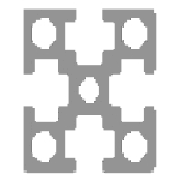
# Autodesk Inventor part: r150
Saved by Autodesk Inventor 2018 (Build 220112000, 112)
## iProperties
_CCFamilyMember: 1
_CCFamilyDisplayName: MISUMI_AFS - MISUMI Frame Family
_FrameMemberDoc: Frame Member File
_Version: 15.0.0
_GetPNFromCC: 1
Created: 2016-02-19
Part Number: r150
Material: アルミニウム 6061
Description: MISUMI Frame Family
Document SubType Name: Modeling
Standard: 名称未設定
Designer: gisen
Language: ja-JP
Size Designation: (名称未設定 1)
Categories: <MemberInstance><Categories><Category DisplayName="形鋼" InternalName="089c4875-fa83-4c05-b084-43b9cc11f5ed" Mnemonic="GRDR"><CategoryParameter DisplayName="長さ単位ごとの質量" InternalName="0bb95a10-148f-4027-a459-38d7b056702a" Mnemonic="shpmass"/><CategoryParameter DisplayName="断面積" InternalName="1ff91680-64b0-4202-b9a3-7fd3f94bba3b" Mnemonic="secarea"/><CategoryParameter DisplayName="回転半径(x)" InternalName="25778675-03e9-40c1-b6a8-4a9ed693320d" Mnemonic="gyrradx"/><CategoryParameter DisplayName="横弾性係数" InternalName="26c1ec35-5026-4c63-ad0a-751cf684a536" Mnemonic="torrigmod"/><CategoryParameter DisplayName="重心 X-X 間の距離" InternalName="26c9bdb8-9c79-4b4f-a92e-8e197583c9c4" Mnemonic="grcendistX"/><CategoryParameter DisplayName="レガシー メンバ ID" InternalName="340afe4f-75d7-48d3-ab7d-943f3c3da468" Mnemonic="LegacyMemberID"/><CategoryParameter DisplayName="基準長さ" InternalName="42e34263-8f20-4d0e-ad48-bf1385b87c24" Mnemonic="shplen"/><CategoryParameter DisplayName="慣性モーメント(y)" InternalName="4b9f58ea-bced-460e-81ea-3d29ca5a49e3" Mnemonic="inermomy"/><CategoryParameter DisplayName="慣性モーメント(x)" InternalName="4cd780bc-73d7-43ac-917a-579e5cbd684d" Mnemonic="inermomx"/><CategoryParameter DisplayName="カスタム基準点" InternalName="4f1d1b73-316d-484b-a3df-9cbabb16eb77" Mnemonic="shpBasePoint"/><CategoryParameter DisplayName="形状の高さ" InternalName="50274e7d-5ac0-4796-92cb-c59e54983c67" Mnemonic="shpheig"/><CategoryParameter DisplayName="断面係数(y)" InternalName="59eaa5e9-d227-48dc-b6c1-6920f96e0f95" Mnemonic="secmody"/><CategoryParameter DisplayName="断面表示記号" InternalName="5a64d034-428d-49c8-ba32-7619764de20f" Mnemonic="shpdes"/><CategoryParameter DisplayName="断面係数(x)" InternalName="72cfad18-cf51-4ed4-aaa7-c6b224f8419f" Mnemonic="secmodx"/><CategoryParameter DisplayName="極断面係数" InternalName="7c55a8dc-8844-49f9-a867-cc677b30ec9a" Mnemonic="torsecmod"/><CategoryParameter DisplayName="形状の幅" InternalName="7c717d54-a18f-4666-b4d4-573cce22c62c" Mnemonic="shpwdth"/><CategoryParameter DisplayName="第二形状の厚さ" InternalName="9251a8e1-85fd-4e47-af99-afdb762317d9" Mnemonic="shpthick2"/><CategoryParameter DisplayName="FG 作成済み" InternalName="9c666724-f362-4ea7-ac62-f6a007de5c69" Mnemonic="shpFGAuto"/><CategoryParameter DisplayName="重心 Y-Y 間の距離" InternalName="bcc4fb17-7af4-436a-8f8c-d0aa3b0248c5" Mnemonic="grcendistY"/><CategoryParameter DisplayName="回転半径(y)" InternalName="bfa18ebe-1636-4dbe-8d42-b263e0b73184" Mnemonic="gyrrady"/><CategoryParameter DisplayName="形状の厚さ" InternalName="d109cf76-8eb4-42fc-9800-4409734adc67" Mnemonic="shpthick"/><CategoryParameter DisplayName="横弾性係数" InternalName="de4c90c6-aaa8-468f-a335-6737b311b5d3" Mnemonic="shdispc"/><Category DisplayName="その他" InternalName="f02205ff-2390-476f-921c-0b3185f88e84" Mnemonic="OTHSHP"><CategoryParameter DisplayName="慣性モーメント(y)" InternalName="044c654e-f649-48ac-84cc-650a29ae31ca" Mnemonic="inermomy"/><CategoryParameter DisplayName="形状の厚さ" InternalName="12b1a788-9233-48fd-a933-2df8ff42b15f" Mnemonic="shpthick"/><CategoryParameter DisplayName="長さ単位ごとの質量" InternalName="2fd289d6-9394-4d2d-97e6-6659d7d4551d" Mnemonic="shpmass"/><CategoryParameter DisplayName="回転半径(y)" InternalName="743e1dfe-1bba-408b-b985-cf752b207386" Mnemonic="gyrrady"/><CategoryParameter DisplayName="断面係数(y)" InternalName="88b8bff9-a616-4028-93d5-ed4f79680d13" Mnemonic="secmody"/><CategoryParameter DisplayName="断面積" InternalName="c46ecdf8-b6eb-4db9-8b25-30258930c1e3" Mnemonic="secarea"/><CategoryParameter DisplayName="断面係数(x)" InternalName="cac70804-9d39-43bb-be17-56ea1f39a6c2" Mnemonic="secmodx"/><CategoryParameter DisplayName="慣性モーメント(x)" InternalName="ec6737bc-264f-43ed-b0bd-f6d410c2718d" Mnemonic="inermomx"/><CategoryParameter DisplayName="回転半径(x)" InternalName="ee72c61e-565e-4fd6-b448-66e1e1abcb7e" Mnemonic="gyrradx"/></Category></Category><Category DisplayName="データタイプ" InternalName="23b78d0f-2648-40c6-8793-ca6db495c9e8" Mnemonic="DATATYPE"><CategoryParameter DisplayName="表示名" InternalName="05415f3d-3907-474b-a020-eb9d644f4cf3" Mnemonic="DISPLAYNAME"/><CategoryParameter DisplayName="規格" InternalName="0c0a119c-1e12-4c84-803f-101930972f5e" Mnemonic="STANDARD"/><CategoryParameter DisplayName="説明" InternalName="13903e3d-64b1-4950-80da-f627842ea37f" Mnemonic="DESCRIPTION"/><CategoryParameter DisplayName="指定" InternalName="2675968c-4ce5-49e0-a4f5-552d29089031" Mnemonic="DESIGNATION"/><CategoryParameter DisplayName="既定行" InternalName="2af9ec52-faaa-4026-b378-f9fa4afca842" Mnemonic="DEFAULTROW"/><CategoryParameter DisplayName="フォルダ名" InternalName="3f06958e-8713-4116-9be7-ed6184ecc97b" Mnemonic="FOLDERNAME"/><CategoryParameter DisplayName="リビジョン ガイド" InternalName="45a75005-10b1-4dfc-8d6d-dfe629f0b93c" Mnemonic="REVISIONGUID"/><CategoryParameter DisplayName="ファイル名" InternalName="8b46a4cc-9585-4fed-90c3-899f57e09a73" Mnemonic="FILENAME"/><CategoryParameter DisplayName="標準化団体" InternalName="8f5914e1-4693-403f-8ab5-d37768198c9d" Mnemonic="STDSORG"/><CategoryParameter DisplayName="ファミリ バージョン" InternalName="914462f6-6e19-4b14-ba84-155b9680b1d0" Mnemonic="FAMILYREVISION"/><CategoryParameter DisplayName="規格のリビジョン" InternalName="91d5a463-65c2-4fde-b823-3b7fea5e8e17" Mnemonic="STANDARDREVISION"/><CategoryParameter DisplayName="メンバ履歴" InternalName="a65d44b9-392f-4f4f-857b-e4b3d54996fe" Mnemonic="MEMBERREVISION"/><CategoryParameter DisplayName="クリップ フォーマット" InternalName="bc51e27b-3422-4e78-93ef-cec197ddf230" Mnemonic="CLIPFORMAT"/><CategoryParameter DisplayName="製造者" InternalName="cd6c7a72-a28a-4e50-99a9-2c7f4e13e5ad" Mnemonic="MANUFACTURER"/><CategoryParameter DisplayName="内部名" InternalName="cf1d0246-76d9-4b4a-8305-fa0409afb5c1" Mnemonic="INTERNALNAME"/><CategoryParameter DisplayName="IsMetric" InternalName="e2385c5b-1ea4-4823-96a8-8de651266ec3" Mnemonic="ISMETRIC"/><Category DisplayName="パーツ" InternalName="c0e0b642-3bcb-4cc8-9e80-f96d35c4afa4" Mnemonic="PART"><CategoryParameter DisplayName="部品番号" InternalName="016b6077-bfbe-49bd-92c9-d8d59c39c941" Mnemonic="PARTNUMBER"/><CategoryParameter DisplayName="ストック番号" InternalName="4dba7c1c-e26c-444e-836c-b08b433409a8" Mnemonic="STOCKNUMBER"/><CategoryParameter DisplayName="材料キー" InternalName="5c9a8adb-dd2b-4535-b97f-0a94a95fe41f" Mnemonic="MATERIALKEY"/><CategoryParameter DisplayName="材料" InternalName="818a152a-d3c3-49ca-80ee-df7d91421b8e" Mnemonic="MATERIAL"/></Category></Category></Categories><FamilyTemplate Id="MISUMI_AFS_2020"><FamilyTemplateParameters><FamilyTemplateParameter ObjectType="kUserParameterObject" ValueType="xs:double" Id="1" ObjectReferenceKey="Length"/><FamilyTemplateParameter ObjectType="kPartComponentDefinitionObject" ValueType="xs:string" Id="4" SubObjectId="Material"/><FamilyTemplateParameter ObjectType="kPropertyObject" ValueType="xs:string" Id="16" ObjectReferenceKey="{32853F0F-3444-11d1-9E93-0060B03C1CA6}" SubObjectId="5"/><FamilyTemplateParameter ObjectType="kPropertyObject" ValueType="xs:string" Id="17" ObjectReferenceKey="{32853F0F-3444-11d1-9E93-0060B03C1CA6}" SubObjectId="52"/></FamilyTemplateParameters></FamilyTemplate><CategoryParameterMap><ParamToTemplateMap><ParamToTemplate CategoryParameter="//CategoryParameter[@InternalName='cf1d0246-76d9-4b4a-8305-fa0409afb5c1']" ConstantValue="a9660291-3f78-4c8b-a635-3bbe41b86f8f"/><ParamToTemplate CategoryParameter="//CategoryParameter[@InternalName='45a75005-10b1-4dfc-8d6d-dfe629f0b93c']" ConstantValue="29fcafd6-0d04-43cc-a0b1-0a0a89f0e392"/><ParamToTemplate CategoryParameter="//CategoryParameter[@InternalName='3f06958e-8713-4116-9be7-ed6184ecc97b']" ConstantValue="MISUMI_AFS"/><ParamToTemplate CategoryParameter="//CategoryParameter[@InternalName='8f5914e1-4693-403f-8ab5-d37768198c9d']" TemplateParameter="9"/><ParamToTemplate CategoryParameter="//CategoryParameter[@InternalName='0c0a119c-1e12-4c84-803f-101930972f5e']" TemplateParameter="10"/><ParamToTemplate CategoryParameter="//CategoryParameter[@InternalName='91d5a463-65c2-4fde-b823-3b7fea5e8e17']" TemplateParameter="11"/><ParamToTemplate CategoryParameter="//CategoryParameter[@InternalName='cd6c7a72-a28a-4e50-99a9-2c7f4e13e5ad']" TemplateParameter="12"/><ParamToTemplate CategoryParameter="//CategoryParameter[@InternalName='13903e3d-64b1-4950-80da-f627842ea37f']" ConstantValue="MISUMI Frame Family"/><ParamToTemplate CategoryParameter="//CategoryParameter[@InternalName='05415f3d-3907-474b-a020-eb9d644f4cf3']" ConstantValue="MISUMI_AFS"/><ParamToTemplate CategoryParameter="//CategoryParameter[@InternalName='914462f6-6e19-4b14-ba84-155b9680b1d0']" ConstantValue="11"/><ParamToTemplate CategoryParameter="//CategoryParameter[@InternalName='bc51e27b-3422-4e78-93ef-cec197ddf230']" ConstantValue="CF_INVENTOR.STDPARTS"/><ParamToTemplate CategoryParameter="//CategoryParameter[@InternalName='e2385c5b-1ea4-4823-96a8-8de651266ec3']" ConstantValue="true"/><ParamToTemplate CategoryParameter="//CategoryParameter[@InternalName='2af9ec52-faaa-4026-b378-f9fa4afca842']" ConstantValue="1"/><ParamToTemplate CategoryParameter="//CategoryParameter[@InternalName='9c666724-f362-4ea7-ac62-f6a007de5c69']" ConstantValue="1"/><ParamToTemplate CategoryParameter="//CategoryParameter[@InternalName='8b46a4cc-9585-4fed-90c3-899f57e09a73']" ConstantValue="MISUMI_AFS_2020-01"/><ParamToTemplate CategoryParameter="//CategoryParameter[@InternalName='a65d44b9-392f-4f4f-857b-e4b3d54996fe']" ConstantValue="ebcc3c34-39b6-4685-9e3f-5186b6460ef6"/><ParamToTemplate CategoryParameter="//CategoryParameter[@InternalName='a65d44b9-392f-4f4f-857b-e4b3d54996fe']" ConstantValue="ebcc3c34-39b6-4685-9e3f-5186b6460ef6"/><ParamToTemplate CategoryParameter="//CategoryParameter[@InternalName='2675968c-4ce5-49e0-a4f5-552d29089031']" TemplateParameter="17"/><ParamToTemplate CategoryParameter="//CategoryParameter[@InternalName='42e34263-8f20-4d0e-ad48-bf1385b87c24']" TemplateParameter="1"/><ParamToTemplate CategoryParameter="//CategoryParameter[@InternalName='818a152a-d3c3-49ca-80ee-df7d91421b8e']" TemplateParameter="4"/><ParamToTemplate CategoryParameter="//CategoryParameter[@InternalName='016b6077-bfbe-49bd-92c9-d8d59c39c941']" TemplateParameter="16"/></ParamToTemplateMap></CategoryParameterMap></MemberInstance>
Mass: 17.0542 g
Surface Area: 58.8805 cm^2
Volume: 6.31635 cm^3
Density: 2.7 g/cm^3
Appearance: アルミニウム - フラット
IsCustomPart: 1
G_L: 150.000 mm
G_W: 20.000 mm
G_H: 20.000 mm
+887DC481-FAB9-4034-909A-FADD795D5F44+CUTDETAIL1: 切り取り
+1932DFA3-DF50-4FE7-AD7F-3E35B646CFDD+CUTDETAIL2: 切り取り
Author: gisen
Autodesk Inventor part; units mm, degrees
ref_plane "YZ Plane" through (0, 0, 0) normal (1, 0, 0) x (0, 1, 0)
ref_plane "XY Plane" through (0, 0, 0) normal (0, 0, 1) x (1, 0, 0)
ref_plane "開始平面" through (0, 0, 0) normal (0, 1, 0) x (-1, 0, 0)
ref_plane "終了平面" through (0, 150, 0) normal (0, 1, 0) x (-1, 0, 0)
sketch "スケッチ" plane through (0, 0, 0) normal (0, 1, 0) x (-1, 0, 0)
  line L0 (8.5, -3.8) -> (8.5, -2.6)
  line L1 (4, -8.3) -> (4, -5)
  circle A0 centre (7, -7) radius 2
  line L2 (10, -2.6) -> (10, -9.5)
  line L3 (2.6, -10) -> (9.5, -10)
  line L4 (2.1, -9.5) -> (2.1, -9)
  line L5 (8.5, -2.1) -> (8.5, -4)
  line L6 (3.8, -4.8) -> (2.6, -4.8)
  line L7 (4.8, -3.8) -> (4.8, -2.6)
  arc A1 (2.1, -4.3) -> (2.6, -4.8) centre (2.6, -4.3) ccw
  arc A2 (2.6, -8.5) -> (2.1, -9) centre (2.6, -9) ccw
  arc A3 (3.8, -8.5) -> (4, -8.3) centre (3.8, -8.3) ccw
  arc A4 (4, -5) -> (3.8, -4.8) centre (3.8, -5) ccw
  arc A5 (2.1, -3.5) -> (1.6, -3) centre (1.6, -3.5) ccw
  arc A6 (2.1, -9.5) -> (2.6, -10) centre (2.6, -9.5) ccw
  arc A7 (9.5, -10) -> (10, -9.5) centre (9.5, -9.5) ccw
  arc A8 (10, -2.6) -> (9.5, -2.1) centre (9.5, -2.6) ccw
  arc A9 (9, -2.1) -> (8.5, -2.6) centre (9, -2.6) ccw
  arc A10 (8.3, -4) -> (8.5, -3.8) centre (8.3, -3.8) ccw
  arc A11 (4.8, -3.8) -> (5, -4) centre (5, -3.8) ccw
  line L8 (4.3, -2.1) -> (3.5, -2.1)
  arc A12 (4.8, -2.6) -> (4.3, -2.1) centre (4.3, -2.6) ccw
  arc A13 (3, -1.6) -> (3.5, -2.1) centre (3.5, -1.6) ccw
  line L9 (2.1, -4.3) -> (2.1, -3.5)
  line L10 (3.8, -8.5) -> (2.6, -8.5)
  line L11 (9.5, -2.1) -> (9, -2.1)
  line L12 (8.3, -4) -> (5, -4)
  circle A14 centre (0, 0) radius 1.65
  arc A15 (8.5, 2.6) -> (9, 2.1) centre (9, 2.6) ccw
  line L13 (8.5, 3.8) -> (8.5, 2.6)
  arc A16 (8.5, 3.8) -> (8.3, 4) centre (8.3, 3.8) ccw
  line L14 (8.3, 4) -> (5, 4)
  line L15 (10, 2.6) -> (10, 9.5)
  arc A17 (10, 9.5) -> (9.5, 10) centre (9.5, 9.5) ccw
  circle A18 centre (7, 7) radius 2
  line L16 (4, 8.3) -> (4, 5)
  line L17 (2.6, 10) -> (9.5, 10)
  line L18 (9.5, 2.1) -> (9, 2.1)
  arc A19 (9.5, 2.1) -> (10, 2.6) centre (9.5, 2.6) ccw
  line L19 (3.8, 8.5) -> (2.6, 8.5)
  line L20 (4.8, 3.8) -> (4.8, 2.6)
  arc A20 (4.3, 2.1) -> (4.8, 2.6) centre (4.3, 2.6) ccw
  line L21 (2.1, 8.5) -> (4, 8.5)
  arc A21 (4, 8.3) -> (3.8, 8.5) centre (3.8, 8.3) ccw
  arc A22 (2.1, 9) -> (2.6, 8.5) centre (2.6, 9) ccw
  arc A23 (2.6, 10) -> (2.1, 9.5) centre (2.6, 9.5) ccw
  line L22 (2.1, 9.5) -> (2.1, 9)
  arc A24 (1.6, 3) -> (2.1, 3.5) centre (1.6, 3.5) ccw
  line L23 (3.8, 4.8) -> (2.6, 4.8)
  arc A25 (5, 4) -> (4.8, 3.8) centre (5, 3.8) ccw
  arc A26 (3.8, 4.8) -> (4, 5) centre (3.8, 5) ccw
  line L24 (4.3, 2.1) -> (3.5, 2.1)
  arc A27 (2.6, 4.8) -> (2.1, 4.3) centre (2.6, 4.3) ccw
  line L25 (2.1, 4.3) -> (2.1, 3.5)
  arc A28 (3.5, 2.1) -> (3, 1.6) centre (3.5, 1.6) ccw
  arc A29 (-2.6, 8.5) -> (-2.1, 9) centre (-2.6, 9) ccw
  line L26 (-3.8, 8.5) -> (-2.6, 8.5)
  arc A30 (-3.8, 8.5) -> (-4, 8.3) centre (-3.8, 8.3) ccw
  line L27 (-4, 8.3) -> (-4, 5)
  line L28 (-2.6, 10) -> (-9.5, 10)
  arc A31 (-9.5, 10) -> (-10, 9.5) centre (-9.5, 9.5) ccw
  circle A32 centre (-7, 7) radius 2
  line L29 (-8.3, 4) -> (-5, 4)
  line L30 (-10, 2.6) -> (-10, 9.5)
  line L31 (-2.1, 9.5) -> (-2.1, 9)
  arc A33 (-2.1, 9.5) -> (-2.6, 10) centre (-2.6, 9.5) ccw
  line L32 (-8.5, 3.8) -> (-8.5, 2.6)
  line L33 (-3.8, 4.8) -> (-2.6, 4.8)
  arc A34 (-2.1, 4.3) -> (-2.6, 4.8) centre (-2.6, 4.3) ccw
  line L34 (-8.5, 2.1) -> (-8.5, 4)
  arc A35 (-8.3, 4) -> (-8.5, 3.8) centre (-8.3, 3.8) ccw
  arc A36 (-9, 2.1) -> (-8.5, 2.6) centre (-9, 2.6) ccw
  arc A37 (-10, 2.6) -> (-9.5, 2.1) centre (-9.5, 2.6) ccw
  line L35 (-9.5, 2.1) -> (-9, 2.1)
  arc A38 (-3, 1.6) -> (-3.5, 2.1) centre (-3.5, 1.6) ccw
  line L36 (-4.8, 3.8) -> (-4.8, 2.6)
  arc A39 (-4, 5) -> (-3.8, 4.8) centre (-3.8, 5) ccw
  arc A40 (-4.8, 3.8) -> (-5, 4) centre (-5, 3.8) ccw
  line L37 (-2.1, 4.3) -> (-2.1, 3.5)
  arc A41 (-4.8, 2.6) -> (-4.3, 2.1) centre (-4.3, 2.6) ccw
  line L38 (-4.3, 2.1) -> (-3.5, 2.1)
  arc A42 (-2.1, 3.5) -> (-1.6, 3) centre (-1.6, 3.5) ccw
  arc A43 (-8.5, -2.6) -> (-9, -2.1) centre (-9, -2.6) ccw
  line L39 (-8.5, -3.8) -> (-8.5, -2.6)
  arc A44 (-8.5, -3.8) -> (-8.3, -4) centre (-8.3, -3.8) ccw
  line L40 (-8.3, -4) -> (-5, -4)
  line L41 (-10, -2.6) -> (-10, -9.5)
  arc A45 (-10, -9.5) -> (-9.5, -10) centre (-9.5, -9.5) ccw
  circle A46 centre (-7, -7) radius 2
  line L42 (-4, -8.3) -> (-4, -5)
  line L43 (-2.6, -10) -> (-9.5, -10)
  line L44 (-9.5, -2.1) -> (-9, -2.1)
  arc A47 (-9.5, -2.1) -> (-10, -2.6) centre (-9.5, -2.6) ccw
  line L45 (-3.8, -8.5) -> (-2.6, -8.5)
  line L46 (-4.8, -3.8) -> (-4.8, -2.6)
  arc A48 (-4.3, -2.1) -> (-4.8, -2.6) centre (-4.3, -2.6) ccw
  line L47 (-2.1, -8.5) -> (-4, -8.5)
  arc A49 (-4, -8.3) -> (-3.8, -8.5) centre (-3.8, -8.3) ccw
  arc A50 (-2.1, -9) -> (-2.6, -8.5) centre (-2.6, -9) ccw
  arc A51 (-2.6, -10) -> (-2.1, -9.5) centre (-2.6, -9.5) ccw
  line L48 (-2.1, -9.5) -> (-2.1, -9)
  arc A52 (-1.6, -3) -> (-2.1, -3.5) centre (-1.6, -3.5) ccw
  line L49 (-3.8, -4.8) -> (-2.6, -4.8)
  arc A53 (-5, -4) -> (-4.8, -3.8) centre (-5, -3.8) ccw
  arc A54 (-3.8, -4.8) -> (-4, -5) centre (-3.8, -5) ccw
  line L50 (-4.3, -2.1) -> (-3.5, -2.1)
  arc A55 (-2.6, -4.8) -> (-2.1, -4.3) centre (-2.6, -4.3) ccw
  line L51 (-2.1, -4.3) -> (-2.1, -3.5)
  arc A56 (-3.5, -2.1) -> (-3, -1.6) centre (-3.5, -1.6) ccw
  line L52 (1.6, -3) -> (-1.6, -3)
  line L53 (-3, -1.6) -> (-3, 1.6)
  line L54 (-1.6, 3) -> (1.6, 3)
  line L55 (3, 1.6) -> (3, -1.6)
  point P0 (2.1, -10)
  point P1 (10, 2.1)
  point P2 (-2.1, 10)
  point P3 (-10, -2.1)
  dimension "d12" = 4
  dimension "d14" = 3.7
  dimension "d16" = 0.5
  dimension "d17" = 0.5
  dimension "d18" = 0.2
  dimension "d19" = 0.5
  dimension "d20" = 0.5
  dimension "d24" = 0.5
  dimension "d25" = 0.2
  dimension "d28" = 0.5
  dimension "d31" = 1.5
  dimension "d36" = 3.7
  dimension "d37" = 1.5
  dimension "d58" = 3.3
  dimension "d65" = 10
  dimension "d67" = 2.1
  dimension "d68" = 2.1
  dimension "d69" = 1.9
  dimension "d70" = 7
  dimension "d72" = 2.1
  dimension "d73" = 2.1
  dimension "d74" = 1.9
  dimension "d75" = 7
  dimension "d76" = 10
  dimension "d80" = 360
  dimension "d82" = 3
  constraints: 112 end point, 104 point on circle, 57 centre point, 20 point on line, 16 tangent, 5 equal radius, 5 horizontal, 4 vertical, 3 perpendicular, 2 coincident, 281 other
  measures "d12" diameter of A0
  measures "d14" distance between parallel lines of L7 L0
  measures "d16" radius of A1
  measures "d17" radius of A2
  measures "d18" radius of A3
  measures "d19" radius of A5
  measures "d20" radius of A6
  measures "d24" radius of A7
  measures "d25" radius of A10
  measures "d28" radius of A12
  measures "d31" distance between parallel lines of L0 L2
  measures "d36" distance between parallel lines of L6 L10
  measures "d37" distance between parallel lines of L10 L3
  measures "d58" diameter of A14
  measures "d65" distance from line of L2 point (0, 0)
  measures "d67" distance from line of L9 point (0, 0)
  measures "d68" distance from line of L4 point (0, 0)
  measures "d69" distance between parallel lines of L1 L4
  measures "d70" horizontal distance of A0.centre point (0, 0)
  measures "d72" distance from line of L8 point (0, 0)
  measures "d73" distance from line of L11 point (0, 0)
  measures "d74" distance between parallel lines of L11 L12
  measures "d75" horizontal distance of A0.centre point (0, 0)
  measures "d76" distance from line of L3 point (0, 0)
  measures "d82" distance from line of L52 point (0, 0)
extrude "ボディ" add sketch "スケッチ" along normal up to surface (150 mm away) from surface at 0
sketch "スケッチ4" plane through (0, 0, 0) normal (0, 1, 0) x (-1, 0, 0)
  line L0 (0, 0) -> (10, 0)
ref_plane "作業平面4" through (0, 0, 0) normal (0, 0, -1) x (-1, 0, 0)
sketch "スケッチ5" plane through (0, 0, 0) normal (0, 0, -1) x (-1, 0, 0)
  line L0 (-2, 0) -> (12, 0)
  line L1 (-2, 150) -> (12, 150)
sketch "スケッチ9" plane through (2.6, 0, -10) normal (0, -1, 0) x (1, 0, 0)
  circle A0 centre (4.4, 3) radius 2 projected
  circle A1 centre (4.4, 17) radius 2 projected
  circle A2 centre (-9.6, 17) radius 2 projected
  circle A3 centre (-9.6, 3) radius 2 projected
  circle A4 centre (-2.6, 10) radius 1.65 projected
  arc A5 (-5.2, 5.2) -> (-4.7, 5.7) centre (-5.2, 5.7) ccw projected
  line L0 (-4.7, 5.7) -> (-4.7, 6.5) projected
  arc A6 (-4.2, 7) -> (-4.7, 6.5) centre (-4.2, 6.5) ccw projected
  line L1 (-4.2, 7) -> (-1, 7) projected
  arc A7 (-0.5, 6.5) -> (-1, 7) centre (-1, 6.5) ccw projected
  line L2 (-0.5, 6.5) -> (-0.5, 5.7) projected
  arc A8 (-0.5, 5.7) -> (0, 5.2) centre (0, 5.7) ccw projected
  line L3 (0, 5.2) -> (1.2, 5.2) projected
  arc A9 (1.4, 5) -> (1.2, 5.2) centre (1.2, 5) ccw projected
  line L4 (1.4, 5) -> (1.4, 1.7) projected
  arc A10 (1.2, 1.5) -> (1.4, 1.7) centre (1.2, 1.7) ccw projected
  line L5 (1.2, 1.5) -> (0, 1.5) projected
  arc A11 (0, 1.5) -> (-0.5, 1) centre (0, 1) ccw projected
  line L6 (-0.5, 1) -> (-0.5, 0.5) projected
  arc A12 (-0.5, 0.5) -> (0, 0) centre (0, 0.5) ccw projected
  line L7 (0, 0) -> (6.9, 0) projected
  arc A13 (6.9, 0) -> (7.4, 0.5) centre (6.9, 0.5) ccw projected
  line L8 (7.4, 0.5) -> (7.4, 7.4) projected
  arc A14 (7.4, 7.4) -> (6.9, 7.9) centre (6.9, 7.4) ccw projected
  line L9 (6.9, 7.9) -> (6.4, 7.9) projected
  arc A15 (6.4, 7.9) -> (5.9, 7.4) centre (6.4, 7.4) ccw projected
  line L10 (5.9, 7.4) -> (5.9, 6.2) projected
  arc A16 (5.7, 6) -> (5.9, 6.2) centre (5.7, 6.2) ccw projected
  line L11 (5.7, 6) -> (2.4, 6) projected
  arc A17 (2.2, 6.2) -> (2.4, 6) centre (2.4, 6.2) ccw projected
  line L12 (2.2, 6.2) -> (2.2, 7.4) projected
  arc A18 (2.2, 7.4) -> (1.7, 7.9) centre (1.7, 7.4) ccw projected
  line L13 (1.7, 7.9) -> (0.9, 7.9) projected
  arc A19 (0.4, 8.4) -> (0.9, 7.9) centre (0.9, 8.4) ccw projected
  line L14 (0.4, 8.4) -> (0.4, 11.6) projected
  arc A20 (0.9, 12.1) -> (0.4, 11.6) centre (0.9, 11.6) ccw projected
  line L15 (0.9, 12.1) -> (1.7, 12.1) projected
  arc A21 (1.7, 12.1) -> (2.2, 12.6) centre (1.7, 12.6) ccw projected
  line L16 (2.2, 12.6) -> (2.2, 13.8) projected
  arc A22 (2.4, 14) -> (2.2, 13.8) centre (2.4, 13.8) ccw projected
  line L17 (2.4, 14) -> (5.7, 14) projected
  arc A23 (5.9, 13.8) -> (5.7, 14) centre (5.7, 13.8) ccw projected
  line L18 (5.9, 13.8) -> (5.9, 12.6) projected
  arc A24 (5.9, 12.6) -> (6.4, 12.1) centre (6.4, 12.6) ccw projected
  line L19 (6.4, 12.1) -> (6.9, 12.1) projected
  arc A25 (6.9, 12.1) -> (7.4, 12.6) centre (6.9, 12.6) ccw projected
  line L20 (7.4, 12.6) -> (7.4, 19.5) projected
  arc A26 (7.4, 19.5) -> (6.9, 20) centre (6.9, 19.5) ccw projected
  line L21 (6.9, 20) -> (0, 20) projected
  arc A27 (0, 20) -> (-0.5, 19.5) centre (0, 19.5) ccw projected
  line L22 (-0.5, 19.5) -> (-0.5, 19) projected
  arc A28 (-0.5, 19) -> (0, 18.5) centre (0, 19) ccw projected
  line L23 (0, 18.5) -> (1.2, 18.5) projected
  arc A29 (1.4, 18.3) -> (1.2, 18.5) centre (1.2, 18.3) ccw projected
  line L24 (1.4, 18.3) -> (1.4, 15) projected
  arc A30 (1.2, 14.8) -> (1.4, 15) centre (1.2, 15) ccw projected
  line L25 (1.2, 14.8) -> (0, 14.8) projected
  arc A31 (0, 14.8) -> (-0.5, 14.3) centre (0, 14.3) ccw projected
  line L26 (-0.5, 14.3) -> (-0.5, 13.5) projected
  arc A32 (-1, 13) -> (-0.5, 13.5) centre (-1, 13.5) ccw projected
  line L27 (-1, 13) -> (-4.2, 13) projected
  arc A33 (-4.7, 13.5) -> (-4.2, 13) centre (-4.2, 13.5) ccw projected
  line L28 (-4.7, 13.5) -> (-4.7, 14.3) projected
  arc A34 (-4.7, 14.3) -> (-5.2, 14.8) centre (-5.2, 14.3) ccw projected
  line L29 (-5.2, 14.8) -> (-6.4, 14.8) projected
  arc A35 (-6.6, 15) -> (-6.4, 14.8) centre (-6.4, 15) ccw projected
  line L30 (-6.6, 15) -> (-6.6, 18.3) projected
  arc A36 (-6.4, 18.5) -> (-6.6, 18.3) centre (-6.4, 18.3) ccw projected
  line L31 (-6.4, 18.5) -> (-5.2, 18.5) projected
  arc A37 (-5.2, 18.5) -> (-4.7, 19) centre (-5.2, 19) ccw projected
  line L32 (-4.7, 19) -> (-4.7, 19.5) projected
  arc A38 (-4.7, 19.5) -> (-5.2, 20) centre (-5.2, 19.5) ccw projected
  line L33 (-5.2, 20) -> (-12.1, 20) projected
  arc A39 (-12.1, 20) -> (-12.6, 19.5) centre (-12.1, 19.5) ccw projected
  line L34 (-12.6, 19.5) -> (-12.6, 12.6) projected
  arc A40 (-12.6, 12.6) -> (-12.1, 12.1) centre (-12.1, 12.6) ccw projected
  line L35 (-12.1, 12.1) -> (-11.6, 12.1) projected
  arc A41 (-11.6, 12.1) -> (-11.1, 12.6) centre (-11.6, 12.6) ccw projected
  line L36 (-11.1, 12.6) -> (-11.1, 13.8) projected
  arc A42 (-10.9, 14) -> (-11.1, 13.8) centre (-10.9, 13.8) ccw projected
  line L37 (-10.9, 14) -> (-7.6, 14) projected
  arc A43 (-7.4, 13.8) -> (-7.6, 14) centre (-7.6, 13.8) ccw projected
  line L38 (-7.4, 13.8) -> (-7.4, 12.6) projected
  arc A44 (-7.4, 12.6) -> (-6.9, 12.1) centre (-6.9, 12.6) ccw projected
  line L39 (-6.9, 12.1) -> (-6.1, 12.1) projected
  arc A45 (-5.6, 11.6) -> (-6.1, 12.1) centre (-6.1, 11.6) ccw projected
  line L40 (-5.6, 11.6) -> (-5.6, 8.4) projected
  arc A46 (-6.1, 7.9) -> (-5.6, 8.4) centre (-6.1, 8.4) ccw projected
  line L41 (-6.1, 7.9) -> (-6.9, 7.9) projected
  arc A47 (-6.9, 7.9) -> (-7.4, 7.4) centre (-6.9, 7.4) ccw projected
  line L42 (-7.4, 7.4) -> (-7.4, 6.2) projected
  arc A48 (-7.6, 6) -> (-7.4, 6.2) centre (-7.6, 6.2) ccw projected
  line L43 (-7.6, 6) -> (-10.9, 6) projected
  arc A49 (-11.1, 6.2) -> (-10.9, 6) centre (-10.9, 6.2) ccw projected
  line L44 (-11.1, 6.2) -> (-11.1, 7.4) projected
  arc A50 (-11.1, 7.4) -> (-11.6, 7.9) centre (-11.6, 7.4) ccw projected
  line L45 (-11.6, 7.9) -> (-12.1, 7.9) projected
  arc A51 (-12.1, 7.9) -> (-12.6, 7.4) centre (-12.1, 7.4) ccw projected
  line L46 (-12.6, 7.4) -> (-12.6, 0.5) projected
  arc A52 (-12.6, 0.5) -> (-12.1, 0) centre (-12.1, 0.5) ccw projected
  line L47 (-12.1, 0) -> (-5.2, 0) projected
  arc A53 (-5.2, 0) -> (-4.7, 0.5) centre (-5.2, 0.5) ccw projected
  line L48 (-4.7, 0.5) -> (-4.7, 1) projected
  arc A54 (-4.7, 1) -> (-5.2, 1.5) centre (-5.2, 1) ccw projected
  line L49 (-5.2, 1.5) -> (-6.4, 1.5) projected
  arc A55 (-6.6, 1.7) -> (-6.4, 1.5) centre (-6.4, 1.7) ccw projected
  line L50 (-6.6, 1.7) -> (-6.6, 5) projected
  arc A56 (-6.4, 5.2) -> (-6.6, 5) centre (-6.4, 5) ccw projected
  line L51 (-6.4, 5.2) -> (-5.2, 5.2) projected
  line L52 (6.9, 20) -> (0, 20) projected
  line L53 (-5.2, 20) -> (0, 20)
  line L54 (7.4, 12.6) -> (7.4, 19.5) projected
  line L55 (7.4, 12.6) -> (7.4, 7.4)
  constraints: 4 end point, 1 horizontal, 1 vertical
extrude "押し出し7" add sketch "スケッチ9" against normal blind 150 contours A1 | A14 L9 A15 L10 A16 L11 A17 L12 A18 L13 A19 L14 A20 L15 A21 L16 A22 L17 A23 L18 A24 L19 A25 L55 | A27 L22 A28 L23 A29 L24 A30 L25 A31 L26 A32 L27 A33 L28 A34 L29 A35 L30 A36 L31 A37 L32 A38 L53
sketch "スケッチ10" plane through (-9.5, 0, 10) normal (0, -1, 0) x (1, 0, 0)
  line L0 (-0.5, -12.6) -> (-0.5, -19.5) construction
  line L1 (0, -20) -> (6.9, -20) construction
  arc A0 (-0.5, -19.5) -> (0, -20) centre (0, -19.5) ccw construction
  line L2 (-0.5, -19.5) -> (-0.5, -20) construction
  line L3 (-0.5, -20) -> (0, -20) construction
  arc A1 (0, 0) -> (-0.5, -0.5) centre (0, -0.5) ccw projected
  arc A2 (19.4953, -19.5681) -> (-0.0681, -0.0047) centre (-0.5, -20) ccw
  line L4 (19, 0) -> (0, 0) projected
  arc A3 (19.5, -0.5) -> (19, 0) centre (19, -0.5) ccw projected
  line L5 (19.5, -19.5) -> (19.5, -0.5) projected
  arc A4 (19, -20) -> (19.5, -19.5) centre (19, -19.5) ccw projected
  point P0 (9.5, -10)
  dimension "d101" = 20
  constraints: 4 end point, 4 point on circle, 2 point on line, 1 centre point, 1 coincident
  measures "d101" radius of A2
extrude "押し出し8" cut sketch "スケッチ10" against normal through all
ref_plane "作業平面7" through (-9.5, 75, -10) normal (0, -1, 0) x (1, 0, 0)
equation "\"d99\" = Length"
equation "\"Length\" = 150"
equation "\"G_OFFSET_START\" = 0"
equation "\"G_OFFSET_END\" = 0"
equation "\"G_L\" = 150"
